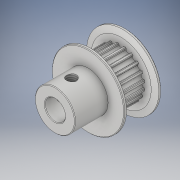
# Autodesk Inventor part: GT2 Belt Pulley
Saved by Autodesk Inventor 2019 (Build 230136000, 136)
## iProperties
Created: 2019-02-09
Part Number: GT2 Belt Pulley
Material: Aluminum
Document SubType Name: Modeling
Designer: Richard Hall
Density: 2.7 g/cm^3
Appearance: Satin
Author: Richard Hall
Autodesk Inventor part; units mm, degrees
ref_plane "YZ Plane" through (0, 0, 0) normal (1, 0, 0) x (0, 1, 0)
ref_plane "XZ Plane" through (0, 0, 0) normal (0, 1, 0) x (-1, 0, 0)
ref_plane "XY Plane" through (0, 0, 0) normal (0, 0, 1) x (1, 0, 0)
sketch "Sketch1" plane through (0, 0, 0) normal (1, 0, 0) x (0, 1, 0)
  line L0 (2.5, 12.875) -> (5, 12.875)
  line L1 (5, 12.875) -> (5, 4.625)
  line L2 (5, 4.625) -> (9, 4.625)
  line L3 (9, 4.625) -> (9, 3.625)
  line L4 (9, 3.625) -> (6, 3.625)
  line L5 (6, 3.625) -> (6, -3.625)
  line L6 (6, -3.625) -> (9, -3.625)
  line L7 (9, -3.625) -> (9, -4.625)
  line L8 (9, -4.625) -> (2.5, -4.625)
  line L9 (2.5, -4.625) -> (2.5, 12.875)
  line L10 (0, 0) -> (0, 5.5243)
  point P0 (6, 0)
  dimension "d0" = 17.5
  dimension "d1" = 2.5
  dimension "d2" = 1
  dimension "d3" = 7.25
  dimension "d5" = 12
  dimension "d6" = 18
  dimension "d7" = 10
  constraints: 22 end point, 8 perpendicular, 2 point on line, 1 collinear, 1 horizontal, 1 horizontal alignment, 1 midpoint, 1 vertical
  measures "d0" distance of L8.end L0.start
  measures "d1" distance from line of L10.start L9
  measures "d2" distance of L6.end L7.end
  measures "d3" distance of L4.end L5.end
  measures "d5" diameter of L5 L10
  measures "d6" diameter of L7 L10
  measures "d7" diameter of L1 L10
revolve "Revolution1" add sketch "Sketch1" angle 360 about axis through (0, 0, 0) along (0, 0, 1)
chamfer "Chamfer1" distance 1.5 angle 15 1 edges at (0, -9, -3.625) measured on face at (0.7179, 7.9128, -3.625)
chamfer "Chamfer2" distance 1.5 angle 15 1 edges at (0, -9, 3.625) measured on face at (1.1966, 7.8547, 3.625)
sketch "Sketch2" plane through (0, 0, -3.625) normal (0, 0, 1) x (1, 0, 0)
  circle A0 centre (0, 0) radius 6 construction
  line L0 (0, 0) -> (-0.9386, 5.9261) construction
  line L1 (0, 0) -> (0.9386, 5.9261) construction
  arc A1 (-0.4989, 5.5618) -> (0.4989, 5.5618) centre (0, 5.805) ccw
  arc A2 (-0.5854, 5.8295) -> (-0.752, 5.9527) centre (-0.7332, 5.8039) ccw
  arc A3 (0.752, 5.9527) -> (0.5854, 5.8295) centre (0.7332, 5.8039) ccw
  arc A4 (-0.5854, 5.8295) -> (-0.4989, 5.5618) centre (0.4, 6) ccw
  arc A5 (0.4989, 5.5618) -> (0.5854, 5.8295) centre (-0.4, 6) ccw
  line L2 (-0.3082, 6) -> (0.256, 6) construction
  line L3 (-0.2283, 5.25) -> (0.3308, 5.25) construction
  arc A6 (0.752, 5.9527) -> (-0.752, 5.9527) centre (0, 0) ccw
  dimension "d15" = 18
  dimension "d16" = 0.555
  dimension "d17" = 0.15
  dimension "d18" = 1
  dimension "d19" = 1
  dimension "d20" = 0.4
  dimension "d21" = 0.4
  dimension "d22" = 0.75
  constraints: 15 point on circle, 8 end point, 6 centre point, 6 tangent, 3 horizontal alignment, 2 equal radius, 2 horizontal, 1 equal length, 1 vertical alignment
  measures "d15" angle of L1 L0
  measures "d16" radius of A1
  measures "d17" radius of A2
  measures "d18" radius of A4
  measures "d19" radius of A5
  measures "d20" horizontal distance of A1.centre A5.centre
  measures "d21" horizontal distance of A4.centre A1.centre
  measures "d22" distance between parallel lines of L3 L2
extrude "Extrusion1" cut sketch "Sketch2" along normal up to surface (7.25 mm away)
pattern_circular "Circular Pattern1" count 20 over 360 about axis through (0, 0, 0) along (0, 0, -1) of "Extrusion1"
sketch "Sketch3" plane through (0, 0, 0) normal (1, 0, 0) x (0, 1, 0)
  line L0 (-5, 4.625) -> (5, 4.625) projected
  line L1 (-5, 12.875) -> (5, 12.875) projected
  point P0 (0, 0)
  point P1 (0, 8.75)
  dimension "d28" = 8.25
  dimension "d29" = 4.125
  constraints: 1 vertical alignment
  measures "d28" distance between parallel lines of L0 L1
  measures "d29" distance from line of point (0, 8.75) L1
hole "Hole1" at (0, 0, 8.75) direction (-1, 0, 0) diameter 2.459 end through all thread size "M3x0.5" class "6H" standard "ANSI Metric M Profile"
pattern_circular "Circular Pattern2" count 2 over 90 about axis through (0, 0, 8.75) along (0, 0, -1) of "Hole1"
chamfer "Chamfer3" distance 0.15 angle 45 5 edges at (0, -5, 12.875) (0, -9, 4.625) (0, -9, -4.625) (0, -2.5, 12.875) (0, -2.5, -4.625)
equation "\"d29\" = 0.5 * d28"
body "Solid1"
